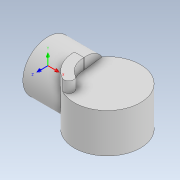
# Autodesk Inventor part: hip_inventor
Saved by Autodesk Inventor 2020 (Build 240168000, 168)
## iProperties
Created: 2021-01-07
Part Number: hip_inventor
Material: Generic
Document SubType Name: Modeling
Designer: DELL
Density: 1 g/cm^3
Appearance: Default
Author: DELL
Autodesk Inventor part; units mm, degrees
ref_plane "YZ Plane" through (0, 0, 0) normal (1, 0, 0) x (0, 1, 0)
ref_plane "XZ Plane" through (0, 0, 0) normal (0, 1, 0) x (-1, 0, 0)
ref_plane "XY Plane" through (0, 0, 0) normal (0, 0, 1) x (1, 0, 0)
sketch "Sketch1" plane through (0, 0, 0) normal (1, 0, 0) x (0, 1, 0)
  circle A0 centre (0, 0) radius 30
  line L0 (-14.5, -26.2631) -> (-14.5, 26.2631)
  line L1 (14.5, -26.2631) -> (14.5, 26.2631)
  line L2 (0, -30) -> (0, 30) construction
  dimension "d0" = 60
  dimension "d19" = 29
  constraints: 6 end point, 6 point on circle, 3 vertical, 1 centre point, 1 coincident, 1 midpoint, 1 other
  measures "d0" diameter of A0
  measures "d19" distance between parallel lines of L1 L0
extrude "Extrusion1" add sketch "Sketch1" along normal blind 71 contours A0 L1 | L0 A0
sketch "Sketch2" plane through (0, 0, 0) normal (0, 1, 0) x (-1, 0, 0)
  line L0 (-71, 26.2631) -> (-71, -26.2631) projected
  circle A0 centre (-71, 0) radius 39.5
  point P0 (0, 0)
  dimension "d3" = 79
  constraints: 1 centre point, 1 midpoint
  measures "d3" diameter of A0
extrude "Extrusion2" add sketch "Sketch2" along normal mid plane 60
sketch "Sketch3" plane through (0, 0, 0) normal (0, 1, 0) x (-1, 0, 0)
  circle A0 centre (-71, 0) radius 39.5 projected
  circle A1 centre (-71, 0) radius 31.5
  circle A2 centre (-71, 0) radius 39.5
  point P0 (0, 0)
  point P1 (-31.5, 0)
  point P2 (-32.9967, 10.7703)
  dimension "d12" = 79
  dimension "d13" = 63
  constraints: 2 centre point, 2 coincident
  measures "d12" diameter of A2
  measures "d13" diameter of A1
sketch "Sketch4" plane through (71, 30, 0) normal (0, 1, 0) x (1, 0, 0)
  circle A0 centre (0, 0) radius 39.5 projected
  circle A1 centre (0, 0) radius 28
  circle A2 centre (-33.75, 0) radius 5.75
  circle A3 centre (-16.875, -29.2284) radius 5.75
  line L0 (0, 0) -> (-16.875, -29.2284) construction
  line L1 (0, 0) -> (-33.75, 0) construction
  line L2 (-23.9531, 26.2631) -> (-26.0362, 26.2631)
  line L3 (-71, 26.2631) -> (-29.5042, 26.2631) projected
  line L4 (-71, 26.2631) -> (-29.5042, 26.2631) projected
  line L5 (-29.5042, 26.2631) -> (-23.9531, 26.2631)
  point P0 (-71, 0)
  point P1 (-39.5, 0)
  point P2 (-71, 0)
  point P3 (-71, 0)
  point P4 (-28, 0)
  point P5 (-14, -24.2487)
  point P6 (-19.75, -34.208)
  point P7 (-34.3715, 23.9531)
  point P8 (-28.0594, 0.824)
  point P9 (-39.5, 0)
  point P10 (-10.7703, 38.0033)
  dimension "d20" = 56
  dimension "d21" = 60
  constraints: 8 end point, 2 centre point, 2 coincident, 2 collinear, 2 horizontal, 2 tangent, 1 horizontal alignment, 1 point on line, 5 other
  measures "d20" diameter of A1
  measures "d21" angle of L1 L0
extrude "Extrusion5" add sketch "Sketch1" along normal up to surface contours L1 A0 L0
extrude "Extrusion3" cut sketch "Sketch4" against normal blind 13 contours A0 A3 A1 A2 | A1 picked at (-5.679, -32.5969)
sketch "Sketch6" plane through (0, 30, 0) normal (0, 1, 0) x (1, 0, 0)
  arc A0 (43, 0) -> (31.5, 0) centre (37.25, 0) ccw projected
  line L0 (40.1901, 24.7184) -> (31.5, 24.7184)
  line L1 (31.5, 24.7184) -> (31.5, 0)
  circle A1 centre (71, 0) radius 39.5 projected
  line L2 (40.1901, 24.7184) -> (42.9622, 0.6581)
  arc A2 (43, 0) -> (31.5, 0) centre (37.25, 0) ccw projected
  arc A3 (43, 0) -> (57, -24.2487) centre (71, 0) ccw projected
  point P0 (0, 0)
  point P1 (42.9622, 0.6581)
  point P2 (71, -39.5)
  point P3 (32.9967, -10.7703)
  point P4 (31.5, 0)
  point P5 (31.5, 0)
  constraints: 6 end point, 2 tangent, 1 coincident, 1 horizontal, 1 perpendicular, 4 other
extrude "Extrusion7" add sketch "Sketch6" against normal up to surface (13 mm away) contours A0 A1 L2 | L1 L0 A1 picked at (39.2874, 16.0263)
sketch "Sketch5" plane through (0, 0, 0) normal (-1, 0, 0) x (0, 0, 1)
  circle A0 centre (0, 0) radius 30 projected
  line L0 (-24.7184, 17) -> (-24.7184, 30)
  line L1 (0, 30) -> (-0.6581, 30) projected
  line L2 (-24.7184, 30) -> (0, 30)
  point P0 (34.208, 17)
  point P1 (39.5, 28)
  point P2 (-8.4816, 28.7761)
  constraints: 4 end point, 1 horizontal, 1 point on circle, 1 vertical
extrude "Extrusion6" cut sketch "Sketch5" against normal through all contours A0 L0 L2 L1
body "Solid1"
